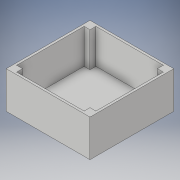
# Autodesk Inventor part: 546-1590YFLBK-3.62x3.62-Enclosure
Saved by Autodesk Inventor 2018 (Build 220112000, 112)
## iProperties
Created: 2018-04-27
Part Number: 546-1590YFLBK-3.62x3.62-Enclosure
Material: Generic
Document SubType Name: Modeling
Designer: bbramman
Density: 1 g/cm^3
Appearance: Default
Author: bbramman
Autodesk Inventor part; units mm, degrees
ref_plane "YZ Plane" through (0, 0, 0) normal (1, 0, 0) x (0, 1, 0)
ref_plane "XZ Plane" through (0, 0, 0) normal (0, 1, 0) x (-1, 0, 0)
ref_plane "XY Plane" through (0, 0, 0) normal (0, 0, 1) x (1, 0, 0)
sketch "Sketch1" plane through (0, 0, 0) normal (0, 1, 0) x (-1, 0, 0)
  line L0 (45.9867, -45.9867) -> (-45.9867, -45.9867)
  line L1 (-45.9867, -45.9867) -> (-45.9867, 45.9867)
  line L2 (-45.9867, 45.9867) -> (45.9867, 45.9867)
  line L3 (45.9867, 45.9867) -> (45.9867, -45.9867)
  line L4 (45.9867, -45.9867) -> (-45.9867, 45.9867) construction
  line L5 (-45.9867, -45.9867) -> (45.9867, 45.9867) construction
  point P0 (0, 0)
  dimension "d0" = 91.9734
  dimension "d1" = 91.9734
  constraints: 12 end point, 2 midpoint, 2 parallel, 1 horizontal, 1 perpendicular
  measures "d0" distance of L1.end L2.end
  measures "d1" distance of L0.end L1.end
extrude "Extrusion1" add sketch "Sketch1" along normal blind 2.4892
sketch "Sketch2" plane through (0, 2.4892, 0) normal (0, 1, 0) x (1, 0, 0)
  line L0 (-45.9867, -45.9867) -> (45.9867, -45.9867) projected
  line L1 (45.9867, 45.9867) -> (-45.9867, 45.9867) projected
  line L2 (-45.9867, -45.9867) -> (45.9867, -45.9867)
  line L3 (45.9867, -45.9867) -> (45.9867, 45.9867)
  line L4 (45.9867, 45.9867) -> (-45.9867, 45.9867)
  line L5 (-45.9867, 45.9867) -> (-45.9867, -45.9867)
  line L6 (43.4975, -43.4975) -> (-43.4975, 43.4975) construction
  line L7 (-43.4975, -43.4975) -> (43.4975, 43.4975) construction
  line L8 (-45.9867, -45.9867) -> (-36.9951, -45.9867)
  line L9 (-45.9867, -36.9951) -> (-45.9867, -45.9867)
  line L10 (-45.9867, 45.9867) -> (-45.9867, -45.9867) projected
  line L11 (-45.9867, 45.9867) -> (-36.9951, 45.9867)
  line L12 (-45.9867, 36.9951) -> (-45.9867, 45.9867)
  line L13 (45.9867, 45.9867) -> (36.9951, 45.9867)
  line L14 (45.9867, 36.9951) -> (45.9867, 45.9867)
  line L15 (45.9867, -45.9867) -> (36.9951, -45.9867)
  line L16 (45.9867, -36.9951) -> (45.9867, -45.9867)
  line L17 (-36.9951, -43.4975) -> (-36.9951, -36.9951)
  line L18 (-36.9951, -36.9951) -> (-43.4975, -36.9951)
  line L19 (-43.4975, 36.9951) -> (-36.9951, 36.9951)
  line L20 (-36.9951, 36.9951) -> (-36.9951, 43.4975)
  line L21 (36.9951, 36.9951) -> (43.4975, 36.9951)
  line L22 (36.9951, 43.4975) -> (36.9951, 36.9951)
  line L23 (43.4975, -36.9951) -> (36.9951, -36.9951)
  line L24 (36.9951, -36.9951) -> (36.9951, -43.4975)
  line L25 (-36.9951, -43.4975) -> (36.9951, -43.4975)
  line L26 (43.4975, -36.9951) -> (43.4975, 36.9951)
  line L27 (36.9951, 43.4975) -> (-36.9951, 43.4975)
  line L28 (-43.4975, 36.9951) -> (-43.4975, -36.9951)
  point P0 (0, 0)
  dimension "d4" = 86.995
  dimension "d5" = 86.995
  dimension "d6" = 8.9916
  dimension "d7" = 8.9916
  dimension "d10" = 8.9916
  dimension "d11" = 8.9916
  constraints: 52 end point, 7 horizontal, 5 perpendicular, 2 midpoint, 2 parallel
  measures "d4" distance of L6.end L7.end
  measures "d5" distance of L7.start L6.end
  measures "d6" distance of L9.start L17.end
  measures "d7" distance of L17.end L8.end
  measures "d10" distance of L14.start L21.start
  measures "d11" distance of L21.start L13.end
extrude "Extrusion2" add sketch "Sketch2" along normal blind 37.9984
body "Solid1"
